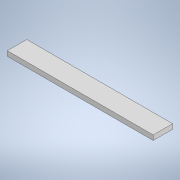
# Autodesk Inventor part: simple_hall
Saved by Autodesk Inventor 2020.2 (Build 242310000, 310)
## iProperties
Created: 2021-03-12
Part Number: simple_hall
Material: Generic
Document SubType Name: Modeling
Designer: Tarsoly
Density: 1 g/cm^3
Appearance: Default
Author: Tarsoly
Autodesk Inventor part; units mm, degrees
ref_plane "YZ Plane" through (0, 0, 0) normal (1, 0, 0) x (0, 1, 0)
ref_plane "XZ Plane" through (0, 0, 0) normal (0, 1, 0) x (-1, 0, 0)
ref_plane "XY Plane" through (0, 0, 0) normal (0, 0, 1) x (1, 0, 0)
sketch "Sketch1" plane through (0, 0, 0) normal (0, 1, 0) x (-1, 0, 0)
  line L0 (2500, 2500) -> (-2500, 2500)
  line L1 (-2500, 2500) -> (-2500, -2500)
  line L2 (-2500, -2500) -> (2500, -2500)
  line L3 (2500, -2500) -> (2500, 2500)
  line L4 (2500, 2500) -> (-2500, -2500) construction
  line L5 (-2500, 2500) -> (2500, -2500) construction
  line L6 (2500, 1000) -> (-500, 1000)
  line L7 (-500, 1000) -> (-500, 600)
  line L8 (-500, 600) -> (2500, 600)
  line L9 (2500, 600) -> (2500, 1000)
  point P0 (0, 0)
  dimension "d0" = 5000
  dimension "d1" = 5000
  dimension "d2" = 3000
  dimension "d3" = 400
  dimension "d4" = 1500
  constraints: 20 end point, 4 parallel, 2 horizontal, 2 midpoint, 2 perpendicular, 1 point on line
  measures "d0" distance of L2.end L1.end
  measures "d1" distance of L1.end L0.end
  measures "d2" distance of L8.end L7.end
  measures "d3" distance of L7.end L6.end
  measures "d4" distance between parallel lines of L0 L6
extrude "Extrusion1" add sketch "Sketch1" along normal blind 100 contours L3 L8 L7 L6
body "Solid1"
